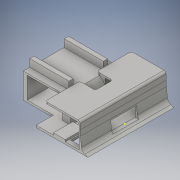
# Autodesk Inventor part: Part1
Saved by Autodesk Inventor 2016 (Build 200138000, 138)
## iProperties
Created: 2015-09-15
Part Number: Part1
Material: Generic
Document SubType Name: Modeling
Designer: cem
Density: 1 g/cm^3
Appearance: Default
Author: cem
Autodesk Inventor part; units mm, degrees
ref_plane "YZ Plane" through (0, 0, 0) normal (1, 0, 0) x (0, 1, 0)
ref_plane "XZ Plane" through (0, 0, 0) normal (0, 1, 0) x (-1, 0, 0)
ref_plane "XY Plane" through (0, 0, 0) normal (0, 0, 1) x (1, 0, 0)
sketch "Sketch1" plane through (0, 0, 0) normal (0, 1, 0) x (-1, 0, 0)
  line L0 (-25.4, 25.4) -> (25.4, 25.4)
  line L1 (25.4, 25.4) -> (25.4, -25.4)
  line L2 (25.4, -25.4) -> (-25.4, -25.4)
  line L3 (-25.4, -25.4) -> (-25.4, 25.4)
  line L4 (-25.4, 25.4) -> (25.4, -25.4) construction
  line L5 (25.4, 25.4) -> (-25.4, -25.4) construction
  line L6 (25.4, 25.4) -> (5.08, 25.4)
  line L7 (5.08, 25.4) -> (5.08, 15.24)
  line L8 (5.08, 15.24) -> (25.4, 15.24)
  line L9 (25.4, 15.24) -> (25.4, 25.4)
  line L10 (25.4, -25.4) -> (0, -25.4)
  line L11 (0, -25.4) -> (0, -15.24)
  line L12 (0, -15.24) -> (25.4, -15.24)
  line L13 (25.4, -15.24) -> (25.4, -25.4)
  point P0 (0, 0)
  dimension "d0" = 50.8
  dimension "d1" = 50.8
  dimension "d2" = 20.32
  dimension "d3" = 10.16
  dimension "d4" = 25.4
  dimension "d5" = 10.16
  constraints: 28 end point, 6 parallel, 3 horizontal, 3 perpendicular, 2 midpoint
  measures "d0" distance of L1.end L2.end
  measures "d1" distance of L0.end L1.end
  measures "d2" distance of L8.end L7.end
  measures "d3" distance of L7.end L6.end
  measures "d4" distance of L11.end L12.end
  measures "d5" distance of L10.end L11.end
extrude "Extrusion1" add sketch "Sketch1" along normal blind 1.27 contours L0 L7 L8 L1 L12 L11 L2 L3
sketch "Sketch2" plane through (0, 1.27, 0) normal (0, 1, 0) x (1, 0, 0)
  line L0 (17.78, -22.86) -> (12.7, -22.86)
  line L1 (12.7, -22.86) -> (12.7, -17.78)
  line L2 (12.7, -17.78) -> (17.78, -17.78)
  line L3 (17.78, -17.78) -> (17.78, -22.86)
  line L4 (25.4, -25.4) -> (25.4, 25.4) projected
  line L5 (-5.08, -25.4) -> (25.4, -25.4) projected
  line L6 (17.78, 22.86) -> (12.7, 22.86)
  line L7 (12.7, 22.86) -> (12.7, 17.78)
  line L8 (12.7, 17.78) -> (17.78, 17.78)
  line L9 (17.78, 17.78) -> (17.78, 22.86)
  line L10 (25.4, 25.4) -> (0, 25.4) projected
  point P0 (0, 0)
  dimension "d8" = 5.08
  dimension "d9" = 5.08
  dimension "d10" = 7.62
  dimension "d11" = 2.54
  dimension "d12" = 5.08
  dimension "d13" = 5.08
  dimension "d14" = 2.54
  constraints: 16 end point, 4 parallel, 2 horizontal, 2 perpendicular
  measures "d8" distance of L1.end L2.end
  measures "d9" distance of L0.end L1.end
  measures "d10" distance from line of L4 L0.start
  measures "d11" distance from line of L5 L0.start
  measures "d12" distance of L8.end L7.end
  measures "d13" distance of L7.end L6.end
  measures "d14" distance from line of L10 L6.start
extrude "Extrusion2" cut sketch "Sketch2" against normal blind 17.78
sketch "Sketch3" plane through (0, 1.27, 0) normal (0, 1, 0) x (1, 0, 0)
  line L0 (-25.4, 15.24) -> (0, 15.24) projected
  line L1 (-5.08, -15.24) -> (-25.4, -15.24) projected
  line L2 (-25.4, 15.24) -> (-5.08, 15.24)
  line L3 (-5.08, 15.24) -> (-5.08, -15.24)
  line L4 (-5.08, -15.24) -> (-25.4, -15.24)
  line L5 (-25.4, -15.24) -> (-25.4, 15.24)
  point P0 (0, 0)
  constraints: 8 end point, 2 parallel, 1 horizontal, 1 perpendicular
extrude "Extrusion3" add sketch "Sketch3" along normal blind 6.35
sketch "Sketch4" plane through (0, 7.62, 0) normal (0, 1, 0) x (1, 0, 0)
  line L0 (-25.4, -15.24) -> (-5.08, -15.24) projected
  line L1 (-20.574, -15.24) -> (-9.906, -15.24)
  line L2 (-9.906, -15.24) -> (-9.906, 15.24)
  line L3 (-9.906, 15.24) -> (-20.574, 15.24)
  line L4 (-20.574, 15.24) -> (-20.574, -15.24)
  line L5 (-25.4, 15.24) -> (-25.4, -15.24) projected
  point P0 (0, 0)
  dimension "d19" = 10.668
  dimension "d20" = 30.48
  dimension "d21" = 4.826
  constraints: 8 end point, 2 parallel, 1 horizontal, 1 perpendicular, 1 point on line
  measures "d19" distance of L3.end L2.end
  measures "d20" distance of L3.end L1.start
  measures "d21" distance from line of L5 L3.end
extrude "Extrusion4" cut sketch "Sketch4" against normal blind 6.35
sketch "Sketch5" plane through (0, 1.27, 0) normal (0, 1, 0) x (1, 0, 0)
  line L0 (-5.08, 15.24) -> (-5.08, -15.24) projected
  line L1 (-5.08, 15.24) -> (7.62, 15.24)
  line L2 (7.62, 15.24) -> (7.62, -15.24)
  line L3 (7.62, -15.24) -> (-5.08, -15.24)
  line L4 (-5.08, -15.24) -> (-5.08, 15.24)
  point P0 (0, 0)
  dimension "d24" = 12.7
  constraints: 8 end point, 2 parallel, 1 horizontal, 1 perpendicular
  measures "d24" distance of L2.end L3.end
extrude "Extrusion5" add sketch "Sketch5" along normal blind 6.35
sketch "Sketch6" plane through (0, 7.62, 0) normal (0, 1, 0) x (1, 0, 0)
  line L0 (-9.906, 15.2776) -> (1.524, 15.2776)
  line L1 (1.524, 15.2776) -> (1.524, -15.2024)
  line L2 (1.524, -15.2024) -> (-9.906, -15.2024)
  line L3 (-9.906, -15.2024) -> (-9.906, 15.2776)
  line L4 (-9.906, 15.24) -> (-9.906, -15.24) projected
  point P0 (0, 0)
  dimension "d27" = 11.43
  dimension "d28" = 30.48
  dimension "d29" = 0
  constraints: 8 end point, 2 parallel, 1 horizontal, 1 perpendicular
  measures "d27" distance of L1.end L2.end
  measures "d28" distance of L0.end L1.end
  measures "d29" distance from line of L4 L0.start
extrude "Extrusion6" cut sketch "Sketch6" against normal blind 6.35
sketch "Sketch7" plane through (-25.4, 0, 15.24) normal (0, 0, 1) x (1, 0, 0)
  line L0 (4.826, 1.27) -> (25.4, 1.27) projected
  line L1 (15.4946, 1.27) -> (28.1946, 1.27)
  line L2 (28.1946, 1.27) -> (28.1946, 297.4869)
  line L3 (28.1946, 297.4869) -> (15.4946, 297.4869)
  line L4 (15.4946, 297.4869) -> (15.4946, 1.27)
  point P0 (25.4, 0)
  dimension "d32" = 12.7
  constraints: 8 end point, 2 parallel, 1 horizontal, 1 perpendicular, 1 point on line
  measures "d32" distance of L3.end L2.end
extrude "Extrusion7" cut sketch "Sketch7" against normal blind 161.925
sketch "Sketch8" plane through (0, 1.27, 0) normal (0, 1, 0) x (1, 0, 0)
  line L0 (-8.7062, 2.1401) -> (-14.2772, 2.1401)
  line L1 (-14.2772, 2.1401) -> (-14.2772, -21.3152)
  line L2 (-14.2772, -21.3152) -> (-8.7062, -21.3152)
  line L3 (-8.7062, -21.3152) -> (-8.7062, 2.1401)
  point P0 (0, 0)
  constraints: 8 end point, 2 parallel, 1 horizontal, 1 perpendicular
extrude "Extrusion8" cut sketch "Sketch8" along normal blind 161.925
sketch "Sketch9" plane through (0, 7.62, 0) normal (0, 1, 0) x (1, 0, 0)
  line L0 (7.62, -15.24) -> (2.7946, -15.24) projected
  line L1 (7.62, 15.24) -> (3.81, 15.24)
  line L2 (3.81, 15.24) -> (3.81, -15.24)
  line L3 (3.81, -15.24) -> (7.62, -15.24)
  line L4 (7.62, -15.24) -> (7.62, 15.24)
  point P0 (0, 0)
  dimension "d37" = 3.81
  constraints: 8 end point, 2 parallel, 1 horizontal, 1 perpendicular, 1 point on line
  measures "d37" distance of L3.end L2.end
extrude "Extrusion9" cut sketch "Sketch9" against normal blind 6.35
sketch "Sketch10" plane through (0, 1.27, 0) normal (0, 1, 0) x (1, 0, 0)
  line L0 (-20.574, 15.24) -> (0, 15.24) projected
  line L1 (25.4, 25.4) -> (0, 25.4) projected
  line L2 (0, 15.24) -> (5.08, 15.24)
  line L3 (5.08, 15.24) -> (5.08, 25.4)
  line L4 (5.08, 25.4) -> (0, 25.4)
  line L5 (0, 25.4) -> (0, 15.24)
  point P0 (0, 0)
  dimension "d40" = 5.08
  constraints: 8 end point, 2 parallel, 1 horizontal, 1 perpendicular, 1 point on line
  measures "d40" distance of L4.end L3.end
extrude "Extrusion10" cut sketch "Sketch10" against normal blind 14.2875
sketch "Sketch11" plane through (0, 1.27, 0) normal (0, 1, 0) x (1, 0, 0)
  line L0 (2.7946, -15.24) -> (2.7946, 15.24) projected
  line L1 (2.7946, 15.24) -> (-20.574, 15.24) projected
  line L2 (2.7946, -15.24) -> (0.2546, -15.24)
  line L3 (0.2546, -15.24) -> (0.2546, 15.24)
  line L4 (0.2546, 15.24) -> (2.7946, 15.24)
  line L5 (2.7946, 15.24) -> (2.7946, -15.24)
  point P0 (0, 0)
  dimension "d43" = 2.54
  constraints: 8 end point, 2 parallel, 1 horizontal, 1 perpendicular, 1 point on line
  measures "d43" distance of L3.end L4.end
extrude "Extrusion11" add sketch "Sketch11" along normal blind 6.35
sketch "Sketch12" plane through (-5.08, 0, 25.4) normal (0, 0, 1) x (1, 0, 0)
  line L0 (0, 1.27) -> (30.48, 1.27) projected
  line L1 (30.48, 1.27) -> (25.4, 1.27)
  line L2 (25.4, 1.27) -> (25.4, 13.97)
  line L3 (25.4, 13.97) -> (30.48, 13.97)
  line L4 (30.48, 13.97) -> (30.48, 1.27)
  point P0 (5.08, 0)
  dimension "d46" = 5.08
  dimension "d47" = 12.7
  constraints: 8 end point, 2 parallel, 1 horizontal, 1 perpendicular
  measures "d46" distance of L2.end L3.end
  measures "d47" distance of L1.end L2.end
extrude "Extrusion12" add sketch "Sketch12" against normal blind 50.8
sketch "Sketch13" plane through (-5.08, 0, 25.4) normal (0, 0, 1) x (1, 0, 0)
  line L0 (30.48, 0) -> (30.48, 13.97) projected
  line L1 (30.48, 0) -> (26.9474, 1.4273)
  line L2 (30.48, 0) -> (34.29, 0) construction
  line L3 (25.4, 1.27) -> (25.4, 13.97) projected
  line L4 (26.9474, 1.4273) -> (25.4, 13.97)
  line L5 (25.4, 13.97) -> (30.48, 13.97)
  point P0 (5.08, 0)
  dimension "d50" = 3.81
  dimension "d51" = 158
  constraints: 8 end point, 1 equal length, 1 horizontal, 1 perpendicular
  measures "d50" distance of L0.start L1.end
  measures "d51" angle of L2 L1
extrude "Extrusion13" cut sketch "Sketch13" against normal blind 68.2625
fillet "Fillet1" radius 3.175 1 edges at (21.8674, 1.4273, 0)
sketch "Sketch14" plane through (-5.08, 0, 25.4) normal (0, 0, 1) x (1, 0, 0)
  line L0 (25.4, 1.27) -> (25.4, 13.97) projected
  line L1 (25.4, 10.16) -> (29.3983, 10.16)
  line L2 (29.3983, 10.16) -> (29.3983, 14.3355)
  line L3 (29.3983, 14.3355) -> (25.4, 14.3355)
  line L4 (25.4, 14.3355) -> (25.4, 10.16)
  line L5 (0, 1.27) -> (25.4, 1.27) projected
  point P0 (5.08, 0)
  dimension "d55" = 8.89
  constraints: 8 end point, 2 parallel, 1 horizontal, 1 perpendicular, 1 point on line
  measures "d55" distance from line of L5 L1.start
extrude "Extrusion14" cut sketch "Sketch14" against normal blind 111.125
sketch "Sketch15" plane through (21.6386, 3.2822, 25.4) normal (0.9924754, 0.1224441, 0) x (0, 0, -1)
  point P0 (25.4, -0.608)
sketch "Sketch16" plane through (-25.4, 0, 15.24) normal (0, 0, 1) x (1, 0, 0)
  point P0 (25.4, 0)
sketch "Sketch17" plane through (20.32, 1.27, -25.4) normal (-1, 0, 0) x (0, 0, 1)
  line L0 (33.02, 0.2648) -> (17.78, 0.2648)
  line L1 (17.78, 0.2648) -> (17.78, 6.6148)
  line L2 (17.78, 6.6148) -> (33.02, 6.6148)
  line L3 (33.02, 6.6148) -> (33.02, 0.2648)
  line L4 (0, 0) -> (0, 8.89) projected
  point P0 (25.4, -1.27)
  dimension "d58" = 15.24
  dimension "d59" = 6.35
  dimension "d60" = 17.78
  constraints: 8 end point, 2 parallel, 1 horizontal, 1 perpendicular
  measures "d58" distance of L1.end L2.end
  measures "d59" distance of L0.end L1.end
  measures "d60" distance from line of L4 L1.end
extrude "Extrusion15" cut sketch "Sketch17" against normal blind 31.75
sketch "Sketch18" plane through (0, 1.27, 0) normal (0, 1, 0) x (1, 0, 0)
  line L0 (20.32, 25.4) -> (5.08, 25.4) projected
  line L1 (5.08, 25.4) -> (12.065, 25.4)
  line L2 (12.065, 25.4) -> (12.065, 15.24)
  line L3 (12.065, 15.24) -> (5.08, 15.24)
  line L4 (5.08, 15.24) -> (5.08, 25.4)
  point P0 (0, 0)
  dimension "d63" = 6.985
  dimension "d64" = 10.16
  constraints: 8 end point, 2 parallel, 1 horizontal, 1 perpendicular
  measures "d63" distance of L2.end L3.end
  measures "d64" distance of L1.end L2.end
extrude "Extrusion16" add sketch "Sketch18" along normal blind 1.143
sketch "Sketch19" plane through (0, 1.27, 0) normal (0, 1, 0) x (1, 0, 0)
  line L0 (12.065, 15.24) -> (5.08, 15.24) projected
  line L1 (12.065, 15.24) -> (5.08, 15.24)
  line L2 (5.08, 15.24) -> (5.08, 13.97)
  line L3 (5.08, 13.97) -> (12.065, 13.97)
  line L4 (12.065, 13.97) -> (12.065, 15.24)
  point P0 (0, 0)
  dimension "d67" = 1.27
  constraints: 8 end point, 2 parallel, 1 horizontal, 1 perpendicular
  measures "d67" distance of L2.end L1.end
extrude "Extrusion17" add sketch "Sketch19" along normal blind 1.143
sketch "Sketch20" plane through (0, 1.27, 0) normal (0, 1, 0) x (1, 0, 0)
  line L0 (12.065, -25.4) -> (5.08, -25.4)
  line L1 (5.08, -25.4) -> (5.08, -13.97)
  line L2 (5.08, -13.97) -> (12.065, -13.97)
  line L3 (12.065, -13.97) -> (12.065, -25.4)
  line L4 (-5.08, -25.4) -> (20.32, -25.4) projected
  line L5 (12.065, 13.97) -> (12.065, 25.4) projected
  line L6 (5.08, 25.4) -> (5.08, 13.97) projected
  point P0 (0, 0)
  dimension "d70" = 11.43
  dimension "d71" = 0
  dimension "d72" = 0
  dimension "d73" = 0
  constraints: 8 end point, 2 parallel, 1 horizontal, 1 perpendicular
  measures "d70" distance of L0.end L1.end
  measures "d71" distance from line of L4 L0.start
  measures "d72" distance from line of L5 L2.end
  measures "d73" distance from line of L6 L0.end
extrude "Extrusion18" add sketch "Sketch20" along normal blind 1.143
sketch "Sketch21" plane through (0, 7.62, 0) normal (0, 1, 0) x (1, 0, 0)
  line L0 (-25.4, 15.24) -> (-25.4, -15.24) projected
  line L1 (-5.08, -15.24) -> (-20.574, -15.24) projected
  line L2 (-25.4, 15.24) -> (-20.574, 15.24)
  line L3 (-20.574, 15.24) -> (-20.574, -15.24)
  line L4 (-20.574, -15.24) -> (-25.4, -15.24)
  line L5 (-25.4, -15.24) -> (-25.4, 15.24)
  point P0 (0, 0)
  constraints: 8 end point, 2 parallel, 1 horizontal, 1 perpendicular
extrude "Extrusion19" add sketch "Sketch21" along normal blind 6.35
sketch "Sketch22" plane through (0, 7.62, 0) normal (0, 1, 0) x (1, 0, 0)
  line L0 (3.81, -15.24) -> (0.2546, -15.24) projected
  line L1 (0.2546, 15.24) -> (3.81, 15.24)
  line L2 (3.81, 15.24) -> (3.81, -15.24)
  line L3 (3.81, -15.24) -> (0.2546, -15.24)
  line L4 (0.2546, -15.24) -> (0.2546, 15.24)
  point P0 (0, 0)
  constraints: 8 end point, 2 parallel, 1 horizontal, 1 perpendicular
extrude "Extrusion20" add sketch "Sketch22" along normal blind 6.35
sketch "Sketch23" plane through (0, 13.97, 0) normal (0, 1, 0) x (1, 0, 0)
  line L0 (-25.4, 15.24) -> (5.08, 15.24) projected
  line L1 (3.81, -15.24) -> (0.2546, -15.24) projected
  line L2 (-25.4, 15.24) -> (3.81, 15.24)
  line L3 (3.81, 15.24) -> (3.81, -15.24)
  line L4 (3.81, -15.24) -> (-25.4, -15.24)
  line L5 (-25.4, -15.24) -> (-25.4, 15.24)
  point P0 (0, 0)
  constraints: 8 end point, 2 parallel, 1 horizontal, 1 perpendicular
extrude "Extrusion21" add sketch "Sketch23" along normal blind 1.016
sketch "Sketch24" plane through (-25.4, 0, 15.24) normal (0, 0, 1) x (1, 0, 0)
  line L0 (0, 14.986) -> (29.21, 14.986) projected
  line L1 (0, 0) -> (2.54, 0)
  line L2 (2.54, 0) -> (2.54, 14.986)
  line L3 (2.54, 14.986) -> (0, 14.986)
  line L4 (0, 14.986) -> (0, 0)
  line L5 (20.32, 0) -> (0, 0) projected
  point P0 (25.4, 0)
  dimension "d82" = 2.54
  dimension "d83" = 0
  constraints: 8 end point, 2 parallel, 1 horizontal, 1 perpendicular, 1 point on line
  measures "d82" distance of L3.end L2.end
  measures "d83" distance from line of L5 L1.start
extrude "Extrusion22" cut sketch "Sketch24" against normal blind 43.434
sketch "Sketch25" plane through (-20.574, 1.27, 15.24) normal (0, 0, 1) x (1, 0, 0)
  line L0 (25.654, 0) -> (24.384, 0) projected
  line L1 (24.384, 13.716) -> (-2.286, 13.716) projected
  line L2 (24.384, 0) -> (22.352, 0)
  line L3 (22.352, 0) -> (22.352, 13.716)
  line L4 (22.352, 13.716) -> (24.384, 13.716)
  line L5 (24.384, 13.716) -> (24.384, 0)
  point P0 (20.574, -1.27)
  dimension "d86" = 2.032
  constraints: 8 end point, 2 parallel, 1 horizontal, 1 perpendicular, 1 point on line
  measures "d86" distance of L3.end L4.end
extrude "Extrusion23" cut sketch "Sketch25" against normal blind 77.216
sketch "Sketch26" plane through (0, 1.27, 0) normal (0, 1, 0) x (1, 0, 0)
  line L0 (0.2546, -15.24) -> (0.2546, 15.24) projected
  line L1 (0.2546, 15.24) -> (5.08, 15.24)
  line L2 (5.08, 15.24) -> (5.08, -15.24)
  line L3 (5.08, -15.24) -> (0.2546, -15.24)
  line L4 (0.2546, -15.24) -> (0.2546, 15.24)
  line L5 (5.08, 25.4) -> (5.08, 13.97) projected
  point P0 (0, 0)
  dimension "d91" = 0
  constraints: 8 end point, 2 parallel, 1 horizontal, 1 perpendicular
  measures "d91" distance from line of L5 L1.end
extrude "Extrusion24" add sketch "Sketch26" along normal blind 16.51
sketch "Sketch27" plane through (0, 17.78, 0) normal (0, 1, 0) x (1, 0, 0)
  line L0 (20.79, 25.4) -> (20.79, -25.4) projected
  line L1 (-5.08, -25.4) -> (5.08, -25.4) projected
  line L2 (20.79, 25.4) -> (0.2668, 25.4)
  line L3 (0.2668, 25.4) -> (0.2668, -25.4)
  line L4 (0.2668, -25.4) -> (20.79, -25.4)
  line L5 (20.79, -25.4) -> (20.79, 25.4)
  point P0 (0, 0)
  dimension "d94" = 20.5232
  constraints: 8 end point, 2 parallel, 1 horizontal, 1 perpendicular, 1 point on line
  measures "d94" distance of L4.end L3.end
extrude "Extrusion25" add sketch "Sketch27" against normal blind 1.27
sketch "Sketch28" plane through (20.32, 10.16, 25.4) normal (0, 1, 0) x (1, 0, 0)
  line L0 (0, 50.8) -> (0.47, 50.8) projected
  line L1 (0, 0) -> (0.47, 0)
  line L2 (0.47, 0) -> (0.47, 50.8)
  line L3 (0.47, 50.8) -> (0, 50.8)
  line L4 (0, 50.8) -> (0, 0)
  point P0 (-20.32, 25.4)
  constraints: 8 end point, 2 parallel, 1 horizontal, 1 perpendicular
extrude "Extrusion26" add sketch "Sketch28" along normal blind 7.62
fillet "Fillet3" radius 25.4 1 edges at (20.79, 10.16, 0)
sketch "Sketch29" plane through (0, 17.78, 0) normal (0, 1, 0) x (1, 0, 0)
  line L0 (20.79, 25.4) -> (0.2668, 25.4) projected
  line L1 (0.2668, -25.4) -> (20.79, -25.4) projected
  line L2 (0.2668, 25.4) -> (20.79, 25.4)
  line L3 (20.79, 25.4) -> (20.79, -25.4)
  line L4 (20.79, -25.4) -> (0.2668, -25.4)
  line L5 (0.2668, -25.4) -> (0.2668, 25.4)
  point P0 (0, 0)
  constraints: 8 end point, 2 parallel, 1 horizontal, 1 perpendicular
extrude "Extrusion27" add sketch "Sketch29" against normal blind 2.54
sketch "Sketch30" plane through (-5.08, 0, 25.4) normal (0, 0, 1) x (1, 0, 0)
  line L0 (25.87, 17.78) -> (25.87, 11.7209) projected
  line L1 (5.3468, 17.78) -> (25.87, 17.78)
  line L2 (25.87, 17.78) -> (25.87, 16.256)
  line L3 (25.87, 16.256) -> (5.3468, 16.256)
  line L4 (5.3468, 16.256) -> (5.3468, 17.78)
  point P0 (5.08, 0)
  dimension "d102" = 1.524
  constraints: 8 end point, 2 parallel, 1 horizontal, 1 perpendicular, 1 point on line
  measures "d102" distance between parallel lines of L3 L1
extrude "Extrusion28" cut sketch "Sketch30" against normal blind 67.31
sketch "Sketch31" plane through (0.2668, 16.256, 25.4) normal (0, 1, 0) x (1, 0, 0)
  line L0 (9.6273, -5.9424) -> (-37.0544, -5.9424)
  line L1 (-37.0544, -5.9424) -> (-37.0544, 56.012)
  line L2 (-37.0544, 56.012) -> (9.6273, 56.012)
  line L3 (9.6273, 56.012) -> (9.6273, -5.9424)
  point P0 (-0.2668, 25.4)
  constraints: 8 end point, 2 parallel, 1 horizontal, 1 perpendicular
extrude "Extrusion29" cut sketch "Sketch31" along normal blind 40.64
sketch "Sketch32" plane through (0.2668, 16.256, 25.4) normal (0, 1, 0) x (1, 0, 0)
  line L0 (-9.7918, 30.48) -> (9.2582, 30.48)
  line L1 (9.2582, 30.48) -> (9.2582, 20.32)
  line L2 (9.2582, 20.32) -> (-9.7918, 20.32)
  line L3 (-9.7918, 20.32) -> (-9.7918, 30.48)
  line L4 (-9.7918, 30.48) -> (9.2582, 20.32) construction
  line L5 (9.2582, 30.48) -> (-9.7918, 20.32) construction
  point P0 (-0.2668, 25.4)
  dimension "d107" = 19.05
  dimension "d108" = 10.16
  constraints: 12 end point, 2 midpoint, 2 parallel, 1 horizontal, 1 perpendicular
  measures "d107" distance of L1.end L2.end
  measures "d108" distance of L0.end L1.end
extrude "Extrusion30" cut sketch "Sketch32" against normal blind 1.27
chamfer "Chamfer1" distance 3.175 angle 45 1 edges at (5.08, 14.986, 0)
fillet "Fillet4" radius 1.27 1 edges at (20.32, 15.24, 0)
fillet "Fillet5" radius 1.27 1 edges at (20.79, 16.256, 0)
fillet "Fillet6" radius 1.27 4 edges at (9.525, 15.748, 5.08) (0.2546, 15.621, 5.08) (0.2546, 15.621, -5.08) (9.525, 15.748, -5.08)
fillet "Fillet7" radius 1.27 2 edges at (0.2668, 15.748, 25.4) (0.2668, 15.748, -25.4)
sketch "Sketch33" plane through (0, 14.986, 0) normal (0, 1, 0) x (1, 0, 0)
  line L0 (-22.86, 15.24) -> (-22.86, -15.24) projected
  line L1 (0.2546, 6.35) -> (0.2546, 15.24) projected
  line L2 (-22.86, 11.43) -> (0.2546, 11.43)
  line L3 (0.2546, 11.43) -> (0.2546, 8.89)
  line L4 (0.2546, 8.89) -> (-22.86, 8.89)
  line L5 (-22.86, 8.89) -> (-22.86, 11.43)
  line L6 (-22.86, -11.43) -> (0.2546, -11.43)
  line L7 (0.2546, -11.43) -> (0.2546, -8.89)
  line L8 (0.2546, -8.89) -> (-22.86, -8.89)
  line L9 (-22.86, -8.89) -> (-22.86, -11.43)
  line L10 (0.2546, 15.24) -> (-22.86, 15.24) projected
  line L11 (-22.86, -15.24) -> (0.2546, -15.24) projected
  point P0 (0, 0)
  dimension "d118" = 2.54
  dimension "d119" = 22.86
  dimension "d120" = 2.54
  dimension "d121" = 3.81
  dimension "d122" = 23.1146
  dimension "d123" = 3.81
  constraints: 16 end point, 4 parallel, 4 point on line, 2 horizontal, 2 perpendicular
  measures "d118" distance of L7.end L6.end
  measures "d119" distance between parallel lines of L6 L2
  measures "d120" distance between parallel lines of L2 L4
  measures "d121" distance between parallel lines of L10 L2
  measures "d122" distance of L6.start L6.end
  measures "d123" distance between parallel lines of L11 L6
extrude "Extrusion31" add sketch "Sketch33" along normal blind 4.445 contours L2 L1 L4 L0 | L8 L7 L6 L0
body "Solid1"
